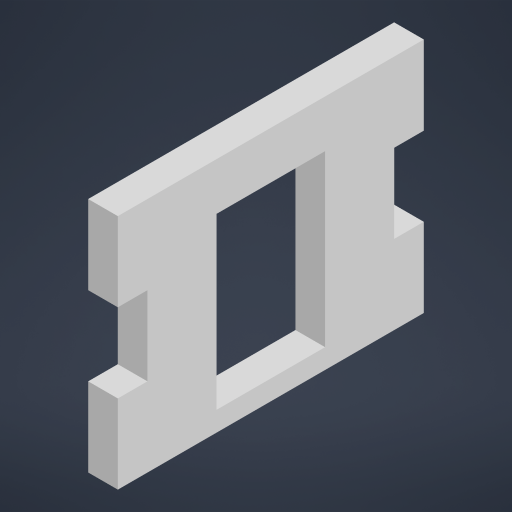
# Autodesk Inventor part: Part1
Saved by Autodesk Inventor 2023 (Build 270158000, 158)
## iProperties
Created: 2023-03-14
Part Number: Part1
Material: Generic
Document SubType Name: Modeling
Designer: Matt
Density: 1 g/cm^3
Appearance: Default
Author: Matt
Autodesk Inventor part; units mm, degrees
ref_plane "YZ Plane" through (0, 0, 0) normal (1, 0, 0) x (0, 1, 0)
ref_plane "XZ Plane" through (0, 0, 0) normal (0, 1, 0) x (-1, 0, 0)
ref_plane "XY Plane" through (0, 0, 0) normal (0, 0, 1) x (1, 0, 0)
sketch "Sketch1" plane through (0, 0, 0) normal (1, 0, 0) x (0, 1, 0)
  line L0 (0, 0) -> (24, 0)
  line L1 (24, 0) -> (24, -25)
  line L2 (24, -25) -> (0, -25)
  line L3 (0, -25) -> (0, 0)
  line L4 (19.2, -7) -> (2, -7)
  line L5 (2, -7) -> (2, -18)
  line L6 (2, -18) -> (19.2, -18)
  line L7 (19.2, -18) -> (19.2, -7)
  line L8 (24, 0) -> (16, 0)
  line L9 (16, 0) -> (16, 3)
  line L10 (16, 3) -> (24, 3)
  line L11 (24, 3) -> (24, 0)
  line L12 (0, 0) -> (8, 0)
  line L13 (8, 0) -> (8, 3)
  line L14 (8, 3) -> (0, 3)
  line L15 (0, 3) -> (0, 0)
  line L16 (0, -12.5) -> (27.6785, -12.5)
  line L17 (24, -25) -> (16, -25)
  line L18 (16, -25) -> (16, -28)
  line L19 (16, -28) -> (24, -28)
  line L20 (24, -28) -> (24, -25)
  line L21 (0, -25) -> (8, -25)
  line L22 (8, -25) -> (8, -28)
  line L23 (8, -28) -> (0, -28)
  line L24 (0, -28) -> (0, -25)
  dimension "d0" = 24
  dimension "d1" = 25
  dimension "d4" = 4.8
  dimension "d5" = 7
  dimension "d6" = 7
  dimension "d7" = 2
  dimension "d8" = 3
  dimension "d9" = 8
  dimension "d10" = 3
  dimension "d11" = 8
  constraints: 50 end point, 8 parallel, 6 symmetric about line, 5 horizontal, 4 perpendicular, 1 midpoint
  measures "d0" distance of L1.end L2.end
  measures "d1" distance of L0.end L1.end
  measures "d4" distance between parallel lines of L1 L7
  measures "d5" distance between parallel lines of L0 L4
  measures "d6" distance between parallel lines of L2 L6
  measures "d7" distance between parallel lines of L3 L5
  measures "d8" distance of L8.end L9.end
  measures "d9" distance of L9.end L10.end
  measures "d10" distance of L12.end L13.end
  measures "d11" distance of L13.end L14.end
extrude "Extrusion1" add sketch "Sketch1" along normal blind 3 contours L15 L14 L13 L0 | L0 L1 L16 L7 L4 L5 L3 | L16 L5 L6 L7 L1 L2 L3 | L9 L10 L11 L0 | L2 L22 L23 L24 | L2 L20 L19 L18
equation "\"d6\" = d5"
equation "\"d9\" = 0.333333 * d0"
equation "\"d10\" = d8"
equation "\"d11\" = 0.333333 * d0"
body "Solid1"
